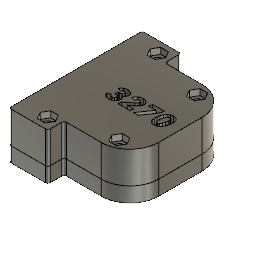
InformerCase (Autodesk Fusion 360 design; units mm, degrees)
Autodesk Fusion 360 part; units mm, degrees
sketch "Main" plane through (0, 0, 0) normal (0, 0, 1) x (1, 0, 0)
  line L0 (0, 0) -> (14.65, 0)
  line L1 (14.65, 0) -> (14.65, 6.955)
  line L2 (14.65, 6.955) -> (32.527, 6.955)
  line L3 (32.527, 6.955) -> (42.842, 17.27)
  line L4 (42.842, 17.27) -> (42.842, 35.76)
  line L5 (42.842, 35.76) -> (32.527, 46.075)
  line L6 (32.527, 46.075) -> (14.65, 46.075)
  line L7 (14.65, 46.075) -> (14.65, 53.03)
  line L8 (14.65, 53.03) -> (0, 53.03)
  line L9 (0, 53.03) -> (0, 0)
  line L10 (0, 26.515) -> (42.842, 26.515) construction
  line L11 (0, 2.995) -> (11.67, 2.995) construction
  line L12 (11.67, 2.995) -> (11.67, 50.035) construction
  line L13 (11.67, 50.035) -> (0, 50.035) construction
  line L14 (0, 50.035) -> (0, 2.995) construction
  line L15 (11.67, 2.995) -> (11.67, 0) construction
  line L16 (11.67, 50.035) -> (11.67, 53.03) construction
  circle A0 centre (11.67, 50.035) radius 1.6
  circle A1 centre (11.67, 2.995) radius 1.6
  line L17 (0, 26.515) -> (35.375, 26.515) construction
  line L18 (35.375, 43.16) -> (35.375, 9.87) construction
  circle A2 centre (35.375, 43.16) radius 1.6
  circle A3 centre (35.375, 9.87) radius 1.6
  line L19 (0, 0) -> (4.1, 0)
  line L20 (4.1, 0) -> (4.1, 53.03)
  line L21 (4.1, 53.03) -> (0, 53.03)
  line L22 (0, 53.03) -> (0, 0)
  line L23 (14.65, 46.075) -> (-0.0168, 46.075)
  line L24 (14.65, 6.955) -> (-0.002, 6.955)
  line L25 (14.65, 46.075) -> (14.65, 6.955)
  line L26 (32.527, 46.075) -> (32.527, 6.955) construction
  line L27 (42.842, 17.27) -> (32.527, 17.27) construction
  line L28 (42.842, 35.76) -> (32.527, 35.76) construction
  arc A4 (42.842, 35.76) -> (32.527, 46.075) centre (32.527, 35.76) ccw
  arc A5 (32.527, 6.955) -> (42.842, 17.27) centre (32.527, 17.27) ccw
  line L29 (13.3154, 47.185) -> (14.9609, 50.035)
  line L30 (14.9609, 50.035) -> (13.3154, 52.885)
  line L31 (13.3154, 52.885) -> (10.0246, 52.885)
  line L32 (10.0246, 52.885) -> (8.3791, 50.035)
  line L33 (8.3791, 50.035) -> (10.0246, 47.185)
  line L34 (10.0246, 47.185) -> (13.3154, 47.185)
  line L35 (10.0227, 5.8439) -> (8.3791, 2.9928)
  line L36 (8.3791, 2.9928) -> (10.0264, 0.1439)
  line L37 (10.0264, 0.1439) -> (13.3173, 0.1461)
  line L38 (13.3173, 0.1461) -> (14.9609, 2.9972)
  line L39 (14.9609, 2.9972) -> (13.3136, 5.8461)
  line L40 (13.3136, 5.8461) -> (10.0227, 5.8439)
  line L41 (33.7279, 12.7191) -> (32.0841, 9.8681)
  line L42 (32.0841, 9.8681) -> (33.7312, 7.0191)
  line L43 (33.7312, 7.0191) -> (37.0221, 7.0209)
  line L44 (37.0221, 7.0209) -> (38.6659, 9.8719)
  line L45 (38.6659, 9.8719) -> (37.0188, 12.7209)
  line L46 (37.0188, 12.7209) -> (33.7279, 12.7191)
  line L47 (33.7284, 46.0093) -> (32.0841, 43.1587)
  line L48 (32.0841, 43.1587) -> (33.7307, 40.3093)
  line L49 (33.7307, 40.3093) -> (37.0216, 40.3107)
  line L50 (37.0216, 40.3107) -> (38.6659, 43.1613)
  line L51 (38.6659, 43.1613) -> (37.0193, 46.0107)
  line L52 (37.0193, 46.0107) -> (33.7284, 46.0093)
  line L53 (39.342, 39.26) -> (39.342, 13.77) construction
  line L54 (39.342, 30.0994) -> (42.842, 30.0994) construction
  circle A6 centre (39.342, 39.26) radius 2.5
  circle A7 centre (39.342, 13.77) radius 2.5
  line L55 (32.527, 46.075) -> (23.027, 46.075)
  line L56 (23.027, 46.075) -> (23.027, 48.075)
  line L57 (23.027, 48.075) -> (32.527, 48.075)
  line L58 (32.527, 48.075) -> (32.527, 46.075)
  line L59 (30, 38.58) -> (30, 14.45) construction
  line L60 (0, 26.515) -> (30, 26.515) construction
  line L61 (31.75, 16.2) -> (28.25, 16.2)
  line L62 (28.25, 16.2) -> (28.25, 12.7)
  line L63 (28.25, 12.7) -> (31.75, 12.7)
  line L64 (31.75, 12.7) -> (31.75, 16.2)
  line L65 (31.75, 16.2) -> (28.25, 12.7) construction
  line L66 (28.25, 16.2) -> (31.75, 12.7) construction
  line L67 (31.75, 36.83) -> (28.25, 36.83)
  line L68 (28.25, 36.83) -> (28.25, 40.33)
  line L69 (28.25, 40.33) -> (31.75, 40.33)
  line L70 (31.75, 40.33) -> (31.75, 36.83)
  line L71 (31.75, 36.83) -> (28.25, 40.33) construction
  line L72 (28.25, 36.83) -> (31.75, 40.33) construction
  line L73 (0, 26.515) -> (35.1, 26.515) construction
  circle A8 centre (35.1, 26.515) radius 1
  line L74 (0, 26.515) -> (31.8, 26.515) construction
  line L75 (31.8, 23.64) -> (31.8, 29.39) construction
  circle A9 centre (31.8, 23.64) radius 1
  circle A10 centre (31.8, 29.39) radius 1
  line L76 (0, 53.03) -> (2.5, 53.03)
  line L77 (2.5, 53.03) -> (2.5, 0)
  line L78 (2.5, 0) -> (0, 0)
  line L79 (0, 0) -> (0, 53.03)
  circle A11 centre (35.1, 26.515) radius 2
  circle A12 centre (31.8, 29.39) radius 2
  circle A13 centre (31.8, 23.64) radius 2
  line L80 (31.25, 15.7) -> (28.75, 15.7)
  line L81 (28.75, 15.7) -> (28.75, 13.2)
  line L82 (28.75, 13.2) -> (31.25, 13.2)
  line L83 (31.25, 13.2) -> (31.25, 15.7)
  line L84 (31.25, 15.7) -> (28.75, 13.2) construction
  line L85 (28.75, 15.7) -> (31.25, 13.2) construction
  line L86 (31.25, 39.83) -> (28.75, 39.83)
  line L87 (28.75, 39.83) -> (28.75, 37.33)
  line L88 (28.75, 37.33) -> (31.25, 37.33)
  line L89 (31.25, 37.33) -> (31.25, 39.83)
  line L90 (31.25, 39.83) -> (28.75, 37.33) construction
  line L91 (28.75, 39.83) -> (31.25, 37.33) construction
  point P0 (11.67, 50.035)
  point P1 (11.67, 2.995)
  point P2 (35.375, 9.87)
  point P3 (35.375, 43.16)
  point P4 (30, 14.45)
  point P5 (30, 38.58)
  point P6 (30, 14.45)
  point P7 (30, 38.58)
  dimension "d1" = 135
  dimension "d2" = 53.03
  dimension "d3" = 6.955
  dimension "d4" = 14.65
  dimension "d6" = 18.49
  dimension "d7" = 11.67
  dimension "d8" = 47.04
  dimension "d11" = 35.375
  dimension "d12" = 33.29
  dimension "d13" = 3.2
  dimension "d14" = 4.1
  dimension "d15" = 42.842
  dimension "d16" = 14.652
  dimension "d45" = 2.85
  dimension "d52" = 3.5
  dimension "d53" = 5
  dimension "d58" = 9.5
  dimension "d66" = 2
  dimension "d67" = 24.13
  dimension "d68" = 30
  dimension "d69" = 3.5
  dimension "d70" = 3.5
  dimension "d74" = 35.1
  dimension "d75" = 2
  dimension "d76" = 31.8
  dimension "d77" = 5.75
  dimension "d81" = 2.5
  dimension "d82" = 4
  dimension "d83" = 2.5
  dimension "d84" = 2.5
  constraint coincident L0.start L9.end
  constraint horizontal L0
  constraint perpendicular L0 L1
  constraint perpendicular L1 L2
  constraint perpendicular L0 L4
  constraint perpendicular L3 L5
  constraint perpendicular L1 L6
  constraint perpendicular L6 L7
  constraint perpendicular L7 L8
  constraint perpendicular L0 L9
  constraint equal L1 L7
  constraint equal L2 L6
  constraint equal L0 L8
  constraint midpoint L9 L10.start
  constraint midpoint L4 L10.end
  constraint horizontal L11
  constraint vertical L12
  constraint horizontal L13
  constraint vertical L14
  constraint coincident L9 L11.start
  constraint coincident L0 L15.end
  constraint perpendicular L0 L15
  constraint coincident L8 L16.end
  constraint perpendicular L8 L16
  constraint equal L15 L16
  constraint coincident P0 L12.end
  constraint coincident P1 L11.end
  constraint perpendicular L14 L17
  constraint vertical L18
  constraint midpoint L17.end L18
  constraint coincident P3 L18.start
  constraint coincident P2 L18.end
  constraint equal A2 A3
  constraint equal A0 A2
  constraint equal A1 A2
  constraint horizontal L19
  constraint vertical L20
  constraint horizontal L21
  constraint vertical L22
  constraint coincident L8 L20.end
  constraint horizontal L23
  constraint horizontal L24
  constraint coincident L26 L27.end
  constraint perpendicular L26 L27
  constraint coincident L26 L28.end
  constraint perpendicular L26 L28
  constraint coincident L5 L53.start
  constraint coincident L3 L53.end
  constraint vertical L53
  constraint coincident L53 L54.start
  constraint coincident L4 L54.end
  constraint perpendicular L4 L54
  constraint coincident L53.start A6.centre
  constraint coincident L53.end A7.centre
  constraint equal A6 A7
  constraint horizontal L55
  constraint vertical L56
  constraint horizontal L57
  constraint vertical L58
  constraint vertical L59
  constraint perpendicular L25 L60
  constraint midpoint L59 L60.end
  constraint perpendicular L61 L62
  constraint parallel L61 L63
  constraint parallel L62 L64
  constraint horizontal L61
  constraint coincident L65 P6
  constraint coincident L66 P6
  constraint coincident P6 P4
  constraint perpendicular L67 L68
  constraint parallel L67 L69
  constraint parallel L68 L70
  constraint horizontal L67
  constraint coincident L71 P7
  constraint coincident L72 P7
  constraint coincident P7 P5
  constraint equal L63 L67
  constraint equal L62 L68
  constraint perpendicular L18 L73
  constraint coincident L73.end A8.centre
  constraint horizontal L74
  constraint vertical L75
  constraint midpoint L74.end L75
  constraint coincident L75.start A9.centre
  constraint coincident L75.end A10.centre
  constraint equal A8 A9
  constraint equal A8 A10
  constraint horizontal L76
  constraint vertical L77
  constraint horizontal L78
  constraint vertical L79
  constraint coincident L0 L77.end
  constraint concentric A8 A11
  constraint concentric A9 A13
  constraint equal A11 A12
  constraint equal A11 A13
  constraint perpendicular L80 L81
  constraint parallel L80 L82
  constraint parallel L81 L83
  constraint horizontal L80
  constraint coincident L84 P6
  constraint coincident L85 P6
  constraint perpendicular L86 L87
  constraint parallel L86 L88
  constraint parallel L87 L89
  constraint horizontal L86
  constraint coincident L90 P7
  constraint coincident L91 P7
  constraint equal L83 L89
  constraint equal L80 L86
  constraint equal L31 L40
  constraint equal L31 L52
  constraint equal L31 L46
  measures "d1" angle of L2 L3
  measures "d2" distance of L0.start L8.end
  measures "d3" distance of L0.end L1.end
  measures "d4" distance of L7.end L8.end
  measures "d6" distance of L3.end L4.end
  measures "d7" distance of P0 L13.end
  measures "d8" distance of L11.start L13.end
  measures "d11" distance of L10.start L17.end
  measures "d12" distance of P3 P2
  measures "d13" diameter of A2
  measures "d14" distance of L0.start L19.end
  measures "d15" distance of L10.start L10.end
  measures "d16" distance of L1.end L24.end
  measures "d45" distance of P0 L34
  measures "d52" distance of L54.start L54.end
  measures "d53" diameter of A6
  measures "d58" distance of L5.end L55.end
  measures "d66" distance of L5.end L57.end
  measures "d67" distance of P7 P6
  measures "d68" distance of L10.start L60.end
  measures "d69" distance of L62.end L63.end
  measures "d70" distance of L61.end L62.end
  measures "d74" distance of L10.start L73.end
  measures "d75" diameter of A8
  measures "d76" distance of L10.start L74.end
  measures "d77" distance of L75.start L75.end
  measures "d81" distance of L8.end L76.end
  measures "d82" diameter of A11
  measures "d83" distance of L81.end L82.end
  measures "d84" distance of L80.start L82.end
extrude "Extrude1" add sketch "Main" along normal blind 3.6 contours L0 L9 L19 L22 L24 L77 L78 L79 | L0 L19 L20 L24 L77 | L9 L22 L23 L24 L77 L79 | L0 L1 L20 L24 L35 L36 L37 L38 L39 L40 | L20 L23 L24 L77 | L8 L9 L21 L22 L23 L76 L77 L79 | L20 L23 L24 L25 | L8 L20 L21 L23 L77 | L1 L35 L36 L37 L38 L39 L40 | L7 L8 L20 L23 L29 L30 L31 L32 L33 L34 | L7 L29 L30 L31 L32 L33 L34 makes body 1
extrude "Extrude2" add sketch "Main" along normal blind 13.48 contours L0 L9 L19 L22 L24 L77 L78 L79 | L0 L19 L20 L24 L77 | L9 L22 L23 L24 L77 L79 | L20 L23 L24 L77 | L8 L9 L21 L22 L23 L76 L77 L79 | L8 L20 L21 L23 L77 bodies 1
extrude "Extrude3" add sketch "Main" along normal blind 10.9 contours L20 L23 L24 L25 bodies 1
extrude "Extrude4" cut sketch "Main" along normal blind 1.6 contours L20 L23 L24 L25 bodies 1
extrude "Extrude5" cut sketch "Main" along normal blind 0.8 contours L0 L9 L19 L22 L24 L77 L78 L79 | L9 L22 L23 L24 L77 L79 | L8 L9 L21 L22 L23 L76 L77 L79 bodies 1
extrude "Extrude6" add sketch "Main" along normal blind 1.6 separate body contours L20 L23 L24 L25 | L2 L3 L4 L5 L6 L25 L41 L42 L45 L46 L47 L48 L49 L50 A6 A7 L55 | L3 A3 L41 L42 L45 L46 | L5 A2 L47 L48 L49 L50 | L3 A7 | L5 A6 | L61 L62 L63 L64 | L67 L68 L69 L70 | A8 | A9 | A10 | A11 | A12 | A13 | L80 L81 L82 L83 | L86 L87 L88 L89 picked at (38.3347, 14.6613) picked at (39.6172, 38.4734) makes body 2
extrude "Extrude7" add sketch "Main" along normal mid plane 20 from surface at 7.2 separate body contours L0 L9 L19 L22 L24 L77 L78 L79 | L0 L19 L20 L24 L77 | L9 L22 L23 L24 L77 L79 | L0 L1 L20 L24 L35 L36 L37 L38 L39 L40 | L20 L23 L24 L77 | L8 L9 L21 L22 L23 L76 L77 L79 | L20 L23 L24 L25 | L8 L20 L21 L23 L77 | L1 L35 L36 L37 L38 L39 L40 | L7 L8 L20 L23 L29 L30 L31 L32 L33 L34 | L2 L3 L4 L5 L6 L25 L41 L42 L45 L46 L47 L48 L49 L50 A6 A7 L55 | L3 A5 L42 | L7 L29 L30 L31 L32 L33 L34 | L3 A3 L41 L42 L45 L46 | L3 A3 A5 L42 L44 L45 | L5 A4 L47 | L3 A3 | L3 A3 | L3 A5 L44 L45 A7 | L5 A2 A4 L47 L50 L51 | L5 A2 L47 L48 L49 L50 | L5 A2 | L5 A2 | L5 A4 L50 L51 A6 | L3 A7 | L3 A7 | L5 A6 | L5 A6 | A0 | A1 | L61 L62 L63 L64 | L67 L68 L69 L70 | A8 | A9 | A10 | A11 | A12 | A13 | L80 L81 L82 L83 | L86 L87 L88 L89 makes body 3
move_face "OffsetFaces1" offset 2 11 faces at (9.7667, 53.03, 3.8667) (14.65, 50.7117, 10.5333) (20.609, 46.075, 10.5333) (37.6845, 44.6931, 10.5333) (42.842, 29.5967, 10.5333) (39.6452, 9.8047, 3.8667) (24.0473, 29.5967, 17.2) (26.568, 6.955, 10.5333) (14.65, 2.3183, 10.5333) (4.8833, 0, 3.8667) (24.0473, 29.5967, -2.8) on bodies 3
shell "Shell1" thickness 2 removed faces 0 bodies 3
extrude "Extrude10" add 1 faces at (26.0473, 29.5967, 19.2) along direction (0, 0, -1) blind 10 on bodies 3 bodies 3
extrude "Extrude9" add sketch "Main" along normal blind 24 from surface at -4.8 contours L0 L9 L19 L22 L24 L77 L78 L79 | L0 L19 L20 L24 L77 | L9 L22 L23 L24 L77 L79 | L0 L1 L20 L24 L35 L36 L37 L38 L39 L40 | L20 L23 L24 L77 | L8 L9 L21 L22 L23 L76 L77 L79 | L8 L20 L21 L23 L77 | L1 L35 L36 L37 L38 L39 L40 | L7 L8 L20 L23 L29 L30 L31 L32 L33 L34 | L7 L29 L30 L31 L32 L33 L34 bodies 3
combine "Combine1" operation cut target body 3 tool bodies 1 keep tools
extrude "Extrude8" cut sketch "Main" along normal mid plane 100 contours L3 A3 | L3 A3 | L5 A2 | L5 A2 | A0 | A1 bodies 3
extrude "Extrude21" cut 1 faces at (22.5007, 31.7006, 19.2) along direction (0, 0, -1) blind 4 on bodies 3 bodies 3
extrude "Extrude11" cut sketch "Main" against normal blind 2.6 from surface at 15.2 contours L1 L35 L36 L37 L38 L39 L40 | L1 L38 L39 | L7 L29 L30 L31 L32 L33 L34 | L7 L29 L30 | L3 A3 L41 L42 L45 L46 | L3 A3 A5 L42 L44 L45 | A5 L42 L43 L44 | L3 A3 | L3 A3 | L5 A2 A4 L47 L50 L51 | L5 A2 L47 L48 L49 L50 | A4 L47 L51 L52 | L5 A2 | L5 A2 | A0 | A1 bodies 3
extrude "Extrude12" add sketch "Main" along normal blind 15 from surface at -2.8 contours L3 A5 L42 | L3 A3 A5 L42 L44 L45 | L5 A4 L47 | L3 A5 L44 L45 A7 | L5 A2 A4 L47 L50 L51 | L5 A4 L50 L51 A6 | L3 A7 | L3 A7 | L5 A6 | L5 A6 bodies 3
combine "Combine2" operation cut target body 3 tool bodies 2 keep tools
extrude "Extrude13" cut sketch "Main" against normal blind 3 contours L6 L55 L56 L57 L58 bodies 3
extrude "Extrude17" cut sketch "Main" against normal blind 20 contours A8 | A9 | A10 bodies 3
fillet "Fillet2" radius 1 3 edges at (30.8677, 29.0284, -4.8) (30.8677, 23.2784, -4.8) (34.1677, 26.1534, -4.8) on bodies 3
chamfer "Chamfer2" distance 2 angle 45 4 edges at (10.1783, 2.4164, -4.8) (10.1783, 49.4564, -4.8) (33.8833, 42.5814, -4.8) (33.8833, 9.2914, -4.8) on bodies 3
fillet "Fillet1" radius 1 6 edges at (16.65, 4.955, 7.2) (16.65, -2, 7.2) (16.65, 48.075, 7.2) (16.65, 55.03, 7.2) (0, 55.03, 7.2) (0, -2, 7.2) on bodies 3
ref_plane "WorkPlane1" through (9.375, 49.5525, 1.6) normal (0, 0, -1) x (-1, 0, 0)
split "Split1" by plane through (9.375, 49.5525, 1.6) normal (0, 0, -1) bodies 3 makes body 4 at (17.5414, 25.656, -4.8)
extrude "Extrude14" cut sketch "Main" along normal up to surface (1.6 mm away) contours L6 L55 L56 L57 L58 bodies 4
extrude "Extrude15" add sketch "Main" along normal up to surface (1.1 mm away) from surface at 0.5 contours L6 L55 L56 L57 L58 bodies 3
extrude "Extrude18" add sketch "Main" against normal blind 2 from surface at -1.5 contours A11 | A12 | A13 bodies 4
sketch "Logo" plane through (0, 0, 0) normal (0, 0, 1) x (1, 0, 0)
  spline S0 degree 3 poles (18.0744, 27.1656) (18.2779, 27.1699) (18.641, 27.1777) (18.9629, 27.3429) (19.1044, 27.4156) knots 0 0 0 0 0.060076 0.107215 0.107215 0.107215 0.107215
  spline S1 degree 3 poles (19.1044, 27.4156) (19.2094, 27.5097) (19.4238, 27.7018) (19.4507, 27.989) (19.4644, 28.1356) knots 0 0 0 0 0.040734 0.083199 0.083199 0.083199 0.083199
  spline S2 degree 3 poles (19.4644, 28.1356) (19.4563, 28.2359) (19.4405, 28.4312) (19.3085, 28.5754) (19.2444, 28.6456) knots 0 0 0 0 0.029271 0.056972 0.056972 0.056972 0.056972
  spline S3 degree 3 poles (19.2444, 28.6456) (19.1637, 28.7009) (18.9896, 28.8204) (18.778, 28.8303) (18.6644, 28.8356) knots 0 0 0 0 0.028776 0.062116 0.062116 0.062116 0.062116
  spline S4 degree 3 poles (18.6644, 28.8356) (18.5409, 28.8289) (18.3029, 28.8161) (18.0946, 28.701) (17.9944, 28.6456) knots 0 0 0 0 0.03656 0.070451 0.070451 0.070451 0.070451
  spline S5 degree 3 poles (17.9944, 28.6456) (17.9082, 28.5777) (17.73, 28.4373) (17.6207, 28.2383) (17.5644, 28.1356) knots 0 0 0 0 0.032575 0.067319 0.067319 0.067319 0.067319
  line L0 (17.5644, 28.1356) -> (16.2244, 28.6756)
  spline S6 degree 3 poles (16.2244, 28.6756) (16.3576, 28.9163) (16.6169, 29.3846) (17.0661, 29.6746) (17.2844, 29.8156) knots 0 0 0 0 0.081125 0.157827 0.157827 0.157827 0.157827
  spline S7 degree 3 poles (17.2844, 29.8156) (17.5216, 29.9206) (18.0026, 30.1335) (18.5281, 30.1614) (18.7944, 30.1756) knots 0 0 0 0 0.07713 0.156393 0.156393 0.156393 0.156393
  spline S8 degree 3 poles (18.7944, 30.1756) (18.9391, 30.1712) (19.2261, 30.1624) (19.5058, 30.0977) (19.6444, 30.0656) knots 0 0 0 0 0.043337 0.085895 0.085895 0.085895 0.085895
  spline S9 degree 3 poles (19.6444, 30.0656) (19.7788, 30.0249) (20.0412, 29.9455) (20.2719, 29.7977) (20.3844, 29.7256) knots 0 0 0 0 0.041908 0.081786 0.081786 0.081786 0.081786
  spline S10 degree 3 poles (20.3844, 29.7256) (20.4859, 29.643) (20.6906, 29.4764) (20.8261, 29.2498) (20.8944, 29.1356) knots 0 0 0 0 0.038931 0.078524 0.078524 0.078524 0.078524
  spline S11 degree 3 poles (20.8944, 29.1356) (20.9527, 29.0093) (21.0755, 28.7431) (21.0879, 28.4498) (21.0944, 28.2956) knots 0 0 0 0 0.041319 0.087093 0.087093 0.087093 0.087093
  spline S12 degree 3 poles (21.0944, 28.2956) (21.0898, 28.1777) (21.0812, 27.9507) (21.0023, 27.7378) (20.9644, 27.6356) knots 0 0 0 0 0.035151 0.067648 0.067648 0.067648 0.067648
  spline S13 degree 3 poles (20.9644, 27.6356) (20.9215, 27.5456) (20.8367, 27.3679) (20.7079, 27.2191) (20.6444, 27.1456) knots 0 0 0 0 0.02975 0.05876 0.05876 0.05876 0.05876
  spline S14 degree 3 poles (20.6444, 27.1456) (20.5759, 27.0791) (20.44, 26.947) (20.2759, 26.8525) (20.1944, 26.8056) knots 0 0 0 0 0.028505 0.056596 0.056596 0.056596 0.056596
  spline S15 degree 3 poles (20.1944, 26.8056) (20.112, 26.7654) (19.9511, 26.6869) (19.7786, 26.639) (19.6944, 26.6156) knots 0 0 0 0 0.027415 0.053588 0.053588 0.053588 0.053588
  line L1 (19.6944, 26.6156) -> (19.6944, 26.5956)
  spline S16 degree 3 poles (19.6944, 26.5956) (19.8543, 26.5394) (20.1682, 26.429) (20.387, 26.1785) (20.4944, 26.0556) knots 0 0 0 0 0.049905 0.097993 0.097993 0.097993 0.097993
  spline S17 degree 3 poles (20.4944, 26.0556) (20.5789, 25.9152) (20.7513, 25.6291) (20.7732, 25.2955) (20.7844, 25.1256) knots 0 0 0 0 0.048411 0.098687 0.098687 0.098687 0.098687
  spline S18 degree 3 poles (20.7844, 25.1256) (20.7762, 24.9353) (20.7605, 24.5703) (20.6143, 24.2358) (20.5444, 24.0756) knots 0 0 0 0 0.056569 0.108536 0.108536 0.108536 0.108536
  spline S19 degree 3 poles (20.5444, 24.0756) (20.4615, 23.9322) (20.2969, 23.6474) (20.048, 23.4324) (19.9244, 23.3256) knots 0 0 0 0 0.049301 0.097922 0.097922 0.097922 0.097922
  spline S20 degree 3 poles (19.9244, 23.3256) (19.7877, 23.2314) (19.509, 23.0391) (19.188, 22.9308) (19.0244, 22.8756) knots 0 0 0 0 0.049528 0.101061 0.101061 0.101061 0.101061
  spline S21 degree 3 poles (19.0244, 22.8756) (18.852, 22.8289) (18.5049, 22.7349) (18.1454, 22.7221) (17.9644, 22.7156) knots 0 0 0 0 0.053367 0.107515 0.107515 0.107515 0.107515
  spline S22 degree 3 poles (17.9644, 22.7156) (17.8061, 22.72) (17.4986, 22.7285) (17.1995, 22.8006) (17.0544, 22.8356) knots 0 0 0 0 0.047345 0.092011 0.092011 0.092011 0.092011
  spline S23 degree 3 poles (17.0544, 22.8356) (16.9187, 22.8762) (16.6522, 22.9559) (16.4122, 23.0965) (16.2944, 23.1656) knots 0 0 0 0 0.042297 0.083121 0.083121 0.083121 0.083121
  spline S24 degree 3 poles (16.2944, 23.1656) (16.1851, 23.247) (15.9657, 23.4105) (15.7983, 23.627) (15.7144, 23.7356) knots 0 0 0 0 0.040686 0.081659 0.081659 0.081659 0.081659
  spline S25 degree 3 poles (15.7144, 23.7356) (15.6418, 23.855) (15.4926, 24.1003) (15.4079, 24.3747) (15.3644, 24.5156) knots 0 0 0 0 0.041741 0.085784 0.085784 0.085784 0.085784
  line L2 (15.3644, 24.5156) -> (16.8844, 24.9256)
  spline S26 degree 3 poles (16.8844, 24.9256) (16.9265, 24.8017) (17.0074, 24.5635) (17.1945, 24.396) (17.2844, 24.3156) knots 0 0 0 0 0.038507 0.07405 0.07405 0.07405 0.07405
  spline S27 degree 3 poles (17.2844, 24.3156) (17.3918, 24.2544) (17.6207, 24.1241) (17.8844, 24.112) (18.0244, 24.1056) knots 0 0 0 0 0.036566 0.077901 0.077901 0.077901 0.077901
  spline S28 degree 3 poles (18.0244, 24.1056) (18.1762, 24.1132) (18.4622, 24.1275) (18.7019, 24.2828) (18.8144, 24.3556) knots 0 0 0 0 0.044689 0.084175 0.084175 0.084175 0.084175
  spline S29 degree 3 poles (18.8144, 24.3556) (18.9048, 24.4489) (19.0909, 24.641) (19.113, 24.9081) (19.1244, 25.0456) knots 0 0 0 0 0.037757 0.077765 0.077765 0.077765 0.077765
  spline S30 degree 3 poles (19.1244, 25.0456) (19.1209, 25.1271) (19.1143, 25.2815) (19.0464, 25.4201) (19.0144, 25.4856) knots 0 0 0 0 0.024157 0.045792 0.045792 0.045792 0.045792
  spline S31 degree 3 poles (19.0144, 25.4856) (18.9777, 25.5423) (18.9044, 25.6556) (18.791, 25.7289) (18.7344, 25.7656) knots 0 0 0 0 0.02 0.04 0.04 0.04 0.04
  spline S32 degree 3 poles (18.7344, 25.7656) (18.6705, 25.7996) (18.5379, 25.8701) (18.3907, 25.9001) (18.3144, 25.9156) knots 0 0 0 0 0.021583 0.044806 0.044806 0.044806 0.044806
  spline S33 degree 3 poles (18.3144, 25.9156) (18.2321, 25.9302) (18.0634, 25.9601) (17.8921, 25.9637) (17.8044, 25.9656) knots 0 0 0 0 0.025032 0.051312 0.051312 0.051312 0.051312
  line L3 (17.8044, 25.9656) -> (17.3644, 25.9656)
  line L4 (17.3644, 25.9656) -> (17.5644, 27.1656)
  line L5 (17.5644, 27.1656) -> (18.0744, 27.1656)
  line L6 (27.1244, 24.3256) -> (26.8744, 22.9056)
  line L7 (26.8744, 22.9056) -> (21.7244, 22.9056)
  line L8 (21.7244, 22.9056) -> (21.9644, 24.2856)
  line L9 (21.9644, 24.2856) -> (25.1544, 26.7756)
  spline S34 degree 3 poles (25.1544, 26.7756) (25.2808, 26.8834) (25.5097, 27.0784) (25.6995, 27.3114) (25.7844, 27.4156) knots 0 0 0 0 0.049727 0.089968 0.089968 0.089968 0.089968
  spline S35 degree 3 poles (25.7844, 27.4156) (25.8485, 27.5098) (25.9704, 27.6888) (25.9934, 27.9037) (26.0044, 28.0056) knots 0 0 0 0 0.033583 0.063837 0.063837 0.063837 0.063837
  spline S36 degree 3 poles (26.0044, 28.0056) (25.997, 28.1143) (25.983, 28.322) (25.8485, 28.4802) (25.7844, 28.5556) knots 0 0 0 0 0.03173 0.060649 0.060649 0.060649 0.060649
  spline S37 degree 3 poles (25.7844, 28.5556) (25.6999, 28.6167) (25.5131, 28.7519) (25.2814, 28.7607) (25.1544, 28.7656) knots 0 0 0 0 0.030612 0.067736 0.067736 0.067736 0.067736
  spline S38 degree 3 poles (25.1544, 28.7656) (25.0199, 28.7548) (24.754, 28.7336) (24.5401, 28.5743) (24.4344, 28.4956) knots 0 0 0 0 0.03958 0.078298 0.078298 0.078298 0.078298
  spline S39 degree 3 poles (24.4344, 28.4956) (24.3427, 28.3951) (24.1463, 28.1799) (24.0537, 27.9031) (24.0044, 27.7556) knots 0 0 0 0 0.040371 0.086429 0.086429 0.086429 0.086429
  line L10 (24.0044, 27.7556) -> (22.5044, 28.0656)
  spline S40 degree 3 poles (22.5044, 28.0656) (22.618, 28.3795) (22.8373, 28.9855) (23.3144, 29.4174) (23.5444, 29.6256) knots 0 0 0 0 0.098444 0.190048 0.190048 0.190048 0.190048
  spline S41 degree 3 poles (23.5444, 29.6256) (23.8079, 29.786) (24.3455, 30.1132) (24.974, 30.1545) (25.2944, 30.1756) knots 0 0 0 0 0.091121 0.185874 0.185874 0.185874 0.185874
  spline S42 degree 3 poles (25.2944, 30.1756) (25.4594, 30.1708) (25.7807, 30.1614) (26.0926, 30.0835) (26.2444, 30.0456) knots 0 0 0 0 0.049357 0.096135 0.096135 0.096135 0.096135
  spline S43 degree 3 poles (26.2444, 30.0456) (26.3845, 29.9981) (26.6572, 29.9056) (26.8908, 29.7374) (27.0044, 29.6556) knots 0 0 0 0 0.044103 0.085847 0.085847 0.085847 0.085847
  spline S44 degree 3 poles (27.0044, 29.6556) (27.1081, 29.5674) (27.3151, 29.3912) (27.448, 29.154) (27.5144, 29.0356) knots 0 0 0 0 0.040492 0.080853 0.080853 0.080853 0.080853
  spline S45 degree 3 poles (27.5144, 29.0356) (27.5698, 28.9083) (27.6849, 28.6437) (27.6977, 28.3552) (27.7044, 28.2056) knots 0 0 0 0 0.041287 0.085791 0.085791 0.085791 0.085791
  spline S46 degree 3 poles (27.7044, 28.2056) (27.7001, 28.0661) (27.6919, 27.8001) (27.6123, 27.5463) (27.5744, 27.4256) knots 0 0 0 0 0.041627 0.079407 0.079407 0.079407 0.079407
  spline S47 degree 3 poles (27.5744, 27.4256) (27.5265, 27.3168) (27.4296, 27.0967) (27.2866, 26.9033) (27.2144, 26.8056) knots 0 0 0 0 0.035556 0.071892 0.071892 0.071892 0.071892
  spline S48 degree 3 poles (27.2144, 26.8056) (27.1366, 26.7093) (26.9777, 26.5123) (26.7902, 26.3424) (26.6944, 26.2556) knots 0 0 0 0 0.037068 0.075792 0.075792 0.075792 0.075792
  spline S49 degree 3 poles (26.6944, 26.2556) (26.5906, 26.1701) (26.3764, 25.9937) (26.1573, 25.8234) (26.0444, 25.7356) knots 0 0 0 0 0.040334 0.083244 0.083244 0.083244 0.083244
  line L11 (26.0444, 25.7356) -> (24.2444, 24.3256)
  line L12 (24.2444, 24.3256) -> (27.1244, 24.3256)
  line L13 (30.3944, 22.9056) -> (28.4044, 22.9056)
  line L14 (28.4044, 22.9056) -> (32.4044, 28.5756)
  line L15 (32.4044, 28.5756) -> (29.1744, 28.5756)
  line L16 (29.1744, 28.5756) -> (29.4144, 29.9856)
  line L17 (29.4144, 29.9856) -> (34.4744, 29.9856)
  line L18 (34.4744, 29.9856) -> (34.2444, 28.6756)
  line L19 (34.2444, 28.6756) -> (30.3944, 22.9056)
  spline S50 degree 3 poles (38.2844, 30.1656) (38.4868, 30.1592) (38.8663, 30.1471) (39.2196, 30.0097) (39.3844, 29.9456) knots 0 0 0 0 0.060251 0.112904 0.112904 0.112904 0.112904
  spline S51 degree 3 poles (39.3844, 29.9456) (39.5286, 29.8717) (39.8084, 29.7284) (40.0213, 29.4974) (40.1244, 29.3856) knots 0 0 0 0 0.048192 0.093453 0.093453 0.093453 0.093453
  spline S52 degree 3 poles (40.1244, 29.3856) (40.2143, 29.2626) (40.3972, 29.0125) (40.4881, 28.7162) (40.5344, 28.5656) knots 0 0 0 0 0.045349 0.092254 0.092254 0.092254 0.092254
  spline S53 degree 3 poles (40.5344, 28.5656) (40.5723, 28.4105) (40.6486, 28.0984) (40.6591, 27.7772) (40.6644, 27.6156) knots 0 0 0 0 0.047756 0.096115 0.096115 0.096115 0.096115
  spline S54 degree 3 poles (40.6644, 27.6156) (40.6606, 27.4437) (40.6529, 27.089) (40.6077, 26.737) (40.5844, 26.5556) knots 0 0 0 0 0.051539 0.106368 0.106368 0.106368 0.106368
  spline S55 degree 3 poles (40.5844, 26.5556) (40.5572, 26.369) (40.5026, 25.9944) (40.4039, 25.629) (40.3544, 25.4456) knots 0 0 0 0 0.056512 0.113447 0.113447 0.113447 0.113447
  spline S56 degree 3 poles (40.3544, 25.4456) (40.2969, 25.2672) (40.1818, 24.9105) (40.0169, 24.5739) (39.9344, 24.4056) knots 0 0 0 0 0.056136 0.11229 0.11229 0.11229 0.11229
  spline S57 degree 3 poles (39.9344, 24.4056) (39.8438, 24.2476) (39.6648, 23.9351) (39.4236, 23.6678) (39.3044, 23.5356) knots 0 0 0 0 0.054458 0.107689 0.107689 0.107689 0.107689
  spline S58 degree 3 poles (39.3044, 23.5356) (39.1747, 23.4181) (38.9125, 23.1805) (38.5949, 23.0245) (38.4344, 22.9456) knots 0 0 0 0 0.052208 0.10558 0.10558 0.10558 0.10558
  spline S59 degree 3 poles (38.4344, 22.9456) (38.262, 22.8815) (37.9042, 22.7482) (37.5223, 22.7333) (37.3244, 22.7256) knots 0 0 0 0 0.054793 0.1138 0.1138 0.1138 0.1138
  spline S60 degree 3 poles (37.3244, 22.7256) (37.1188, 22.7317) (36.734, 22.7431) (36.3727, 22.8744) (36.2044, 22.9356) knots 0 0 0 0 0.061225 0.114602 0.114602 0.114602 0.114602
  spline S61 degree 3 poles (36.2044, 22.9356) (36.0624, 23.0094) (35.7861, 23.1531) (35.5696, 23.3768) (35.4644, 23.4856) knots 0 0 0 0 0.047635 0.092741 0.092741 0.092741 0.092741
  spline S62 degree 3 poles (35.4644, 23.4856) (35.3742, 23.607) (35.1925, 23.8517) (35.094, 24.1402) (35.0444, 24.2856) knots 0 0 0 0 0.045069 0.090843 0.090843 0.090843 0.090843
  spline S63 degree 3 poles (35.0444, 24.2856) (35.0064, 24.4415) (34.9297, 24.757) (34.9195, 25.0815) (34.9144, 25.2456) knots 0 0 0 0 0.048001 0.097108 0.097108 0.097108 0.097108
  spline S64 degree 3 poles (34.9144, 25.2456) (34.9176, 25.4199) (34.9241, 25.7777) (34.964, 26.1333) (34.9844, 26.3156) knots 0 0 0 0 0.052279 0.10728 0.10728 0.10728 0.10728
  spline S65 degree 3 poles (34.9844, 26.3156) (35.0147, 26.504) (35.075, 26.8791) (35.1814, 27.244) (35.2344, 27.4256) knots 0 0 0 0 0.057176 0.113878 0.113878 0.113878 0.113878
  spline S66 degree 3 poles (35.2344, 27.4256) (35.2944, 27.6057) (35.4133, 27.9624) (35.5812, 28.2989) (35.6644, 28.4656) knots 0 0 0 0 0.056858 0.112664 0.112664 0.112664 0.112664
  spline S67 degree 3 poles (35.6644, 28.4656) (35.7572, 28.6255) (35.939, 28.9387) (36.1843, 29.2052) (36.3044, 29.3356) knots 0 0 0 0 0.055279 0.108292 0.108292 0.108292 0.108292
  spline S68 degree 3 poles (36.3044, 29.3356) (36.433, 29.4557) (36.691, 29.6967) (37.0062, 29.8558) (37.1644, 29.9356) knots 0 0 0 0 0.052498 0.105337 0.105337 0.105337 0.105337
  spline S69 degree 3 poles (37.1644, 29.9356) (37.339, 30.0027) (37.6995, 30.1411) (38.0854, 30.1572) (38.2844, 30.1656) knots 0 0 0 0 0.055737 0.115016 0.115016 0.115016 0.115016
  spline S70 degree 3 poles (38.1544, 28.8056) (38.0348, 28.7909) (37.7841, 28.7602) (37.5938, 28.593) (37.4944, 28.5056) knots 0 0 0 0 0.035306 0.074016 0.074016 0.074016 0.074016
  spline S71 degree 3 poles (37.4944, 28.5056) (37.3992, 28.3939) (37.1973, 28.1568) (37.0646, 27.8748) (36.9944, 27.7256) knots 0 0 0 0 0.043809 0.093015 0.093015 0.093015 0.093015
  spline S72 degree 3 poles (36.9944, 27.7256) (36.9274, 27.5603) (36.788, 27.2162) (36.7066, 26.8539) (36.6644, 26.6656) knots 0 0 0 0 0.0534 0.111185 0.111185 0.111185 0.111185
  spline S73 degree 3 poles (36.6644, 26.6656) (36.6323, 26.4702) (36.5687, 26.0827) (36.5591, 25.6902) (36.5544, 25.4956) knots 0 0 0 0 0.059326 0.117641 0.117641 0.117641 0.117641
  spline S74 degree 3 poles (36.5544, 25.4956) (36.5558, 25.4021) (36.5586, 25.2213) (36.5827, 25.0421) (36.5944, 24.9556) knots 0 0 0 0 0.028018 0.05419 0.05419 0.05419 0.05419
  spline S75 degree 3 poles (36.5944, 24.9556) (36.6123, 24.8763) (36.6468, 24.7242) (36.7128, 24.5831) (36.7444, 24.5156) knots 0 0 0 0 0.024317 0.046606 0.046606 0.046606 0.046606
  spline S76 degree 3 poles (36.7444, 24.5156) (36.7825, 24.4589) (36.8572, 24.348) (36.9627, 24.2658) (37.0144, 24.2256) knots 0 0 0 0 0.02035 0.039847 0.039847 0.039847 0.039847
  spline S77 degree 3 poles (37.0144, 24.2256) (37.0747, 24.1935) (37.1997, 24.1271) (37.3412, 24.1195) (37.4144, 24.1156) knots 0 0 0 0 0.020256 0.041931 0.041931 0.041931 0.041931
  spline S78 degree 3 poles (37.4144, 24.1156) (37.5305, 24.1297) (37.7735, 24.1592) (37.958, 24.3211) (38.0544, 24.4056) knots 0 0 0 0 0.034276 0.071736 0.071736 0.071736 0.071736
  spline S79 degree 3 poles (38.0544, 24.4056) (38.1488, 24.5164) (38.348, 24.75) (38.4767, 25.0289) (38.5444, 25.1756) knots 0 0 0 0 0.043458 0.091652 0.091652 0.091652 0.091652
  spline S80 degree 3 poles (38.5444, 25.1756) (38.6108, 25.3408) (38.7492, 25.6845) (38.825, 26.0472) (38.8644, 26.2356) knots 0 0 0 0 0.053313 0.110917 0.110917 0.110917 0.110917
  spline S81 degree 3 poles (38.8644, 26.2356) (38.8994, 26.4326) (38.9693, 26.8262) (38.9793, 27.2259) (38.9844, 27.4256) knots 0 0 0 0 0.05993 0.119755 0.119755 0.119755 0.119755
  spline S82 degree 3 poles (38.9844, 27.4256) (38.9825, 27.5166) (38.9788, 27.6946) (38.9489, 27.87) (38.9344, 27.9556) knots 0 0 0 0 0.027279 0.0533 0.0533 0.0533 0.0533
  spline S83 degree 3 poles (38.9344, 27.9556) (38.9197, 28.0368) (38.8921, 28.1896) (38.8255, 28.3299) (38.7944, 28.3956) knots 0 0 0 0 0.024622 0.046353 0.046353 0.046353 0.046353
  spline S84 degree 3 poles (38.7944, 28.3956) (38.762, 28.4552) (38.6987, 28.5719) (38.5951, 28.655) (38.5444, 28.6956) knots 0 0 0 0 0.020114 0.039403 0.039403 0.039403 0.039403
  spline S85 degree 3 poles (38.5444, 28.6956) (38.4865, 28.7277) (38.3654, 28.7948) (38.2268, 28.8019) (38.1544, 28.8056) knots 0 0 0 0 0.019574 0.041001 0.041001 0.041001 0.041001
  line L20 (15.3141, 26.059) -> (42.0878, 26.059)
  line L21 (42.0878, 26.059) -> (42.0878, 27.059)
  line L22 (42.0878, 27.059) -> (15.3141, 27.059)
  line L23 (15.3141, 27.059) -> (15.3141, 26.059)
  dimension "d101" = 1
  constraint horizontal L20
  constraint vertical L21
  constraint horizontal L22
  constraint vertical L23
  measures "d101" distance of L20.start L22.end
extrude "Extrude22" cut sketch "Logo" against normal blind 8 from surface at 15.2 contours S0 S1 S2 S3 S4 S5 L0 S6 S7 S8 S9 S10 S11 S12 S13 S14 L4 L5 L22 | S14 S15 L1 S16 L4 L20 L22 | S16 S17 S18 S19 S20 S21 S22 S23 S24 S25 L2 S26 S27 S28 S29 S30 S31 S32 S33 L3 L4 L20 | L9 S34 S47 S48 S49 L20 L22 | S34 S35 S36 S37 S38 S39 L10 S40 S41 S42 S43 S44 S45 S46 S47 L22 | L6 L7 L8 L9 S49 L11 L12 L20 | L14 L19 L20 L22 | L14 L15 L16 L17 L18 L19 L22 | L13 L14 L19 L20 | S64 S65 S72 S73 L20 L22 | S50 S51 S52 S53 S54 S65 S66 S67 S68 S69 S70 S71 S72 S81 S82 S83 S84 S85 L22 | S55 S56 S57 S58 S59 S60 S61 S62 S63 S64 S73 S74 S75 S76 S77 S78 S79 S80 L20 | S54 S55 S80 S81 L20 L22 bodies 3 makes body 5 at (38.1982, 26.7845, 9.2)
extrude "Extrude23" add sketch "Logo" against normal up to surface (4 mm away) from surface at 13.2 contours S14 S15 L1 S16 L4 L20 L22 | L4 L20 L22 L23 | S14 S15 L1 S16 L9 S34 L20 L22 | L9 S34 S47 S48 S49 L20 L22 | S47 S48 S49 L14 L20 L22 | L14 L19 L20 L22 | L19 S64 S65 L20 L22 | S64 S65 S72 S73 L20 L22 | S54 S55 S80 S81 L20 L22 | S54 S55 L20 L21 L22 bodies 3 5
extrude "Extrude24" add sketch "Main" against normal blind 2 draft -14 from surface at -2.8 separate body contours L61 L62 L63 L64 | L67 L68 L69 L70 | L80 L81 L82 L83 | L86 L87 L88 L89 makes body 6 at (30.5833, 13.8667, -2.8) makes body 7 at (30.5833, 39.1633, -2.8)
extrude "Extrude25" add sketch "Main" against normal blind 3 from surface at -2.8 contours L80 L81 L82 L83 | L86 L87 L88 L89 bodies 6 7
fillet "Fillet4" radius 1 16 edges at (31.5007, 12.9493, -3.8) (31.25, 13.2, -5.3) (31.25, 15.7, -5.3) (31.5007, 15.9507, -3.8) (28.75, 13.2, -5.3) (28.4993, 12.9493, -3.8) (28.75, 15.7, -5.3) (28.4993, 15.9507, -3.8) (28.75, 37.33, -5.3) (28.4993, 37.0793, -3.8) (28.75, 39.83, -5.3) (28.4993, 40.0807, -3.8) (31.25, 37.33, -5.3) (31.5007, 37.0793, -3.8) (31.25, 39.83, -5.3) (31.5007, 40.0807, -3.8) on bodies 6 7
combine "Combine4" operation cut target body 4 tool bodies 6 7 keep tools
move_face "OffsetFaces3" offset -0.2 16 faces at (28.4162, 14.5437, -3.4667) (29.3032, 16.0303, -3.4671) (30.0937, 16.0338, -3.4667) (31.5803, 15.1468, -3.4671) (31.5838, 14.3563, -3.4667) (31.5803, 13.7532, -3.4671) (30.0937, 12.8662, -3.4667) (29.5111, 13.0334, -4.1338) (29.5111, 37.1634, -4.1338) (28.4162, 38.4863, -3.4667) (28.4197, 39.2768, -3.4671) (29.9063, 40.1638, -3.4667) (31.5803, 39.2768, -3.4671) (31.5838, 38.6737, -3.4667) (30.4889, 37.1634, -4.1338) (30.0937, 36.9962, -3.4667) on bodies 4
move_face "OffsetFaces4" offset -0.2 2 faces at (23.027, 46.7417, 0.8667) (32.527, 46.7417, 1.2333) on bodies 3
hidden bodies 1 2
equation "d3 = ( ( 53.03 - 39.12 ) / 2 ) * 1 mm"
named bodies: "Connector", "Board", "CaseTop", "CaseBottom", "CaseTop (1)", "CaseButton1", "CaseButton2"
